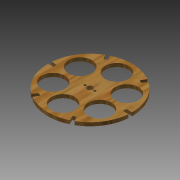
# Autodesk Inventor part: carousel-rev2
Saved by Autodesk Inventor 2013 (Build 170138000, 138)
## iProperties
Created: 2013-07-24
Part Number: carousel-rev2
Material: Generic
Document SubType Name: Modeling
Designer: dkboone
Density: 1 g/cm^3
Mass: 61.9673 g
Surface Area: 287.21 cm^2
Volume: 61.9673 cm^3
Author: dkboone
Autodesk Inventor part; units mm, degrees
ref_plane "YZ Plane" through (0, 0, 0) normal (1, 0, 0) x (0, 1, 0)
ref_plane "XZ Plane" through (0, 0, 0) normal (0, 1, 0) x (-1, 0, 0)
ref_plane "XY Plane" through (0, 0, 0) normal (0, 0, 1) x (1, 0, 0)
sketch "Sketch1" plane through (0, 0, 0) normal (0, 1, 0) x (-1, 0, 0)
  circle A0 centre (0, -48.85) radius 21
  line L0 (0, -48.85) -> (0, 0) construction
  circle A1 centre (42.3053, -24.425) radius 21
  circle A2 centre (42.3053, 24.425) radius 21
  circle A3 centre (0, 48.85) radius 21
  circle A4 centre (-42.3053, 24.425) radius 21
  circle A5 centre (-42.3053, -24.425) radius 21
  circle A6 centre (0, 0) radius 76.2
  circle A7 centre (0, 0) radius 5.08
  dimension "d0" = 42
  dimension "d2" = 48.85
  dimension "d5" = 360
  dimension "d7" = 152.4
  dimension "d8" = 10.16
  constraints: 8 centre point, 2 coincident, 2 end point, 1 vertical, 13 other
  measures "d0" diameter of A0
  measures "d2" distance of L0.start L0.end
  measures "d7" diameter of A6
  measures "d8" diameter of A7
extrude "Extrusion1" add sketch "Sketch1" along normal blind 6.35
sketch "Sketch2" plane through (0, 6.35, 0) normal (0, 1, 0) x (1, 0, 0)
  circle A0 centre (0, 0) radius 5.08 projected
  line L0 (-8.89, 0) -> (8.89, 0) construction
  dimension "d11" = 17.78
  constraints: 2 end point, 1 coincident, 1 horizontal, 1 midpoint
  measures "d11" distance of L0.start L0.end
hole "Hole1" at (-8.89, 6.35, 0) at (8.89, 6.35, 0) direction (0, -1, 0) diameter 4.3053 end through all
sketch "Sketch3" plane through (0, 6.35, 0) normal (0, 1, 0) x (1, 0, 0)
  circle A0 centre (-8.89, 0) radius 2.1526 projected
  circle A1 centre (0, 0) radius 5.08 projected
  circle A2 centre (0, 0) radius 76.2 projected
  line L0 (0, 0) -> (-8.89, 0) construction
  line L1 (-43.1, 74.6514) -> (-33.1, 57.3309)
  arc A3 (-36.4297, 78.1237) -> (-43.1, 74.6514) centre (0, 0) ccw
  arc A4 (-27.9773, 59.9976) -> (-33.1, 57.3309) centre (0, 0) ccw
  line L2 (-36.4297, 78.1237) -> (-27.9773, 59.9976)
  point P0 (-38.1, 65.9911)
  dimension "d30" = 60
  dimension "d35" = 20
  dimension "d37" = 20
  dimension "d38" = 65
  constraints: 7 end point, 4 point on circle, 2 centre point, 1 horizontal, 1 midpoint, 1 point on line, 4 other
  measures "d30" angle of L0 L1
  measures "d35" distance of L1.start L1.end
  measures "d37" distance of L2.end L2.start
  measures "d38" angle of L2 L0
extrude "Extrusion2" cut sketch "Sketch3" against normal through all contours L2 A4 L1 A2 | A2 L1 A3 L2 picked at (-32.0375, 65.438)
pattern_circular "Circular Pattern1" count 6 over 360 about axis through (0, -10, 0) along (0, 1, 0) of "Extrusion2"
equation "\"d37\" = d35"
body "Solid1"
